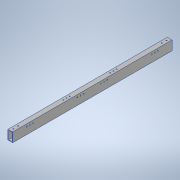
# Autodesk Inventor part: オムニ_角柱4
Saved by Autodesk Inventor 2021 (Build 250183000, 183)
## iProperties
Created: 2021-12-02
Part Number: オムニ_角柱4
Material: アルミニウム 6061
Document SubType Name: Modeling
Designer: 堀川皓史
Density: 2.7 g/cm^3
Appearance: アルミニウム - フラット
Author: 堀川皓史
Autodesk Inventor part; units mm, degrees
ref_plane "YZ Plane" through (0, 0, 0) normal (1, 0, 0) x (0, 1, 0)
ref_plane "XZ Plane" through (0, 0, 0) normal (0, 1, 0) x (-1, 0, 0)
ref_plane "XY Plane" through (0, 0, 0) normal (0, 0, 1) x (1, 0, 0)
sketch "スケッチ1" plane through (0, 0, 0) normal (0, 0, 1) x (1, 0, 0)
  line L0 (7.5, 15) -> (-7.5, 15)
  line L1 (-7.5, 15) -> (-7.5, -15)
  line L2 (-7.5, -15) -> (7.5, -15)
  line L3 (7.5, -15) -> (7.5, 15)
  line L4 (7.5, 15) -> (-7.5, -15) construction
  line L5 (-7.5, 15) -> (7.5, -15) construction
  line L6 (-5.5, 13) -> (5.5, 13)
  line L7 (5.5, 13) -> (5.5, -13)
  line L8 (5.5, -13) -> (-5.5, -13)
  line L9 (-5.5, -13) -> (-5.5, 13)
  point P0 (0, 0)
  dimension "d0" = 15
  dimension "d1" = 30
  dimension "d2" = 2
  constraints: 20 end point, 4 parallel, 2 midpoint, 2 perpendicular, 1 horizontal, 3 other
  measures "d0" distance of L2.end L1.end
  measures "d1" distance of L1.end L0.end
  measures "d2" distance between parallel lines of L0 L6
extrude "押し出し1" add sketch "スケッチ1" along normal blind 510
sketch "スケッチ2" plane through (-7.5, 15, 0) normal (0, 1, 0) x (1, 0, 0)
  circle A0 centre (7.5, -10) radius 1.6
  circle A1 centre (7.5, -25) radius 1.6
  line L0 (15, 0) -> (0, 0) projected
  circle A2 centre (7.5, -500) radius 1.6
  circle A3 centre (7.5, -485) radius 1.6
  line L1 (15, -510) -> (0, -510) projected
  circle A4 centre (7.5, -170) radius 1.6
  circle A5 centre (7.5, -180) radius 1.6
  circle A6 centre (7.5, -190) radius 1.6
  circle A7 centre (7.5, -320) radius 1.6
  circle A8 centre (7.5, -330) radius 1.6
  circle A9 centre (7.5, -340) radius 1.6
  point P0 (7.5, 0)
  point P1 (7.5, 0)
  point P2 (7.5, -510)
  dimension "d5" = 3.2
  dimension "d6" = 3.2
  dimension "d7" = 10
  dimension "d8" = 15
  dimension "d9" = 3.2
  dimension "d10" = 3.2
  dimension "d11" = 10
  dimension "d12" = 15
  dimension "d15" = 3.2
  dimension "d16" = 3.2
  dimension "d17" = 3.2
  dimension "d18" = 10
  dimension "d19" = 10
  dimension "d20" = 180
  dimension "d21" = 3.2
  dimension "d22" = 3.2
  dimension "d23" = 3.2
  dimension "d24" = 10
  dimension "d25" = 10
  dimension "d26" = 180
  constraints: 10 centre point, 10 vertical alignment, 2 midpoint
  measures "d5" diameter of A0
  measures "d6" diameter of A1
  measures "d7" distance of point (7.5, 0) A0.centre
  measures "d8" distance of A0.centre A1.centre
  measures "d9" diameter of A2
  measures "d10" diameter of A3
  measures "d11" distance from line of A2.centre L1
  measures "d12" distance of A3.centre A2.centre
  measures "d15" diameter of A4
  measures "d16" diameter of A5
  measures "d17" diameter of A6
  measures "d18" distance of A5.centre A4.centre
  measures "d19" distance of A6.centre A5.centre
  measures "d20" distance of point (7.5, 0) A5.centre
  measures "d21" diameter of A7
  measures "d22" diameter of A8
  measures "d23" diameter of A9
  measures "d24" distance of A8.centre A7.centre
  measures "d25" distance of A9.centre A8.centre
  measures "d26" distance of point (7.5, -510) A8.centre
extrude "押し出し2" cut sketch "スケッチ2" against normal through all
sketch "スケッチ3" plane through (7.5, -15, 0) normal (1, 0, 0) x (0, 0, -1)
  circle A0 centre (-293, 22.5) radius 1.6
  circle A1 centre (-283, 22.5) radius 1.6
  circle A2 centre (-303, 22.5) radius 1.6
  circle A3 centre (-217, 22.5) radius 1.6
  circle A4 centre (-207, 22.5) radius 1.6
  circle A5 centre (-227, 22.5) radius 1.6
  line L0 (-510, 0) -> (-510, 30) projected
  line L1 (0, 30) -> (-510, 30) projected
  circle A6 centre (-465, 22.5) radius 1.6
  circle A7 centre (-455, 22.5) radius 1.6
  circle A8 centre (-445, 22.5) radius 1.6
  circle A9 centre (-65, 22.5) radius 1.6
  circle A10 centre (-55, 22.5) radius 1.6
  circle A11 centre (-45, 22.5) radius 1.6
  point P0 (0, 15)
  dimension "d27" = 3.2
  dimension "d28" = 3.2
  dimension "d29" = 3.2
  dimension "d30" = 10
  dimension "d31" = 10
  dimension "d32" = 3.2
  dimension "d33" = 3.2
  dimension "d34" = 3.2
  dimension "d35" = 10
  dimension "d36" = 10
  dimension "d37" = 207
  dimension "d38" = 207
  dimension "d39" = 7.5
  dimension "d40" = 7.5
  dimension "d43" = 3.2
  dimension "d44" = 3.2
  dimension "d45" = 3.2
  dimension "d46" = 10
  dimension "d47" = 10
  dimension "d48" = 45
  dimension "d49" = 3.2
  dimension "d50" = 3.2
  dimension "d51" = 3.2
  dimension "d52" = 10
  dimension "d53" = 10
  dimension "d54" = 45
  constraints: 12 centre point, 10 horizontal alignment
  measures "d27" diameter of A0
  measures "d28" diameter of A1
  measures "d29" diameter of A2
  measures "d30" distance of A0.centre A2.centre
  measures "d31" distance of A1.centre A0.centre
  measures "d32" diameter of A3
  measures "d33" diameter of A4
  measures "d34" diameter of A5
  measures "d35" distance of A3.centre A5.centre
  measures "d36" distance of A4.centre A3.centre
  measures "d37" distance from line of L0 A2.centre
  measures "d38" horizontal distance of point (0, 15) A4.centre
  measures "d39" distance from line of L1 A4.centre
  measures "d40" distance from line of L1 A2.centre
  measures "d43" diameter of A6
  measures "d44" diameter of A7
  measures "d45" diameter of A8
  measures "d46" distance of A7.centre A6.centre
  measures "d47" distance of A8.centre A7.centre
  measures "d48" distance from line of L0 A6.centre
  measures "d49" diameter of A9
  measures "d50" diameter of A10
  measures "d51" diameter of A11
  measures "d52" distance of A10.centre A9.centre
  measures "d53" distance of A11.centre A10.centre
  measures "d54" horizontal distance of point (0, 15) A11.centre
extrude "押し出し3" cut sketch "スケッチ3" against normal through all
